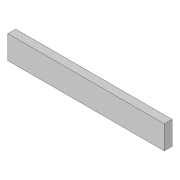
# Autodesk Inventor part: tunnel_line
Saved by Autodesk Inventor 2018 (Build 220112000, 112)
## iProperties
Created: 2017-11-14
Part Number: tunnel_line
Material: Generic
Document SubType Name: Modeling
Designer: Platform
Density: 1 g/cm^3
Appearance: Default
Author: Platform
Autodesk Inventor part; units mm, degrees
ref_plane "YZ Plane" through (0, 0, 0) normal (1, 0, 0) x (0, 1, 0)
ref_plane "XZ Plane" through (0, 0, 0) normal (0, 1, 0) x (-1, 0, 0)
ref_plane "XY Plane" through (0, 0, 0) normal (0, 0, 1) x (1, 0, 0)
sketch "Sketch1" plane through (0, 0, 0) normal (0, 0, 1) x (1, 0, 0)
  line L0 (0, 0) -> (0, 15)
  line L1 (0, 15) -> (100, 15)
  line L2 (100, 15) -> (100, 0)
  line L3 (100, 0) -> (0, 0)
  dimension "d0" = 15
  dimension "d1" = 100
  dimension "d2" = 15
  constraints: 8 end point, 2 perpendicular, 1 vertical
  measures "d0" distance of L0.start L0.end
  measures "d1" distance of L0.end L1.end
  measures "d2" distance of L1.end L2.end
extrude "Extrusion1" add sketch "Sketch1" along normal blind 5
body "Solid1"
